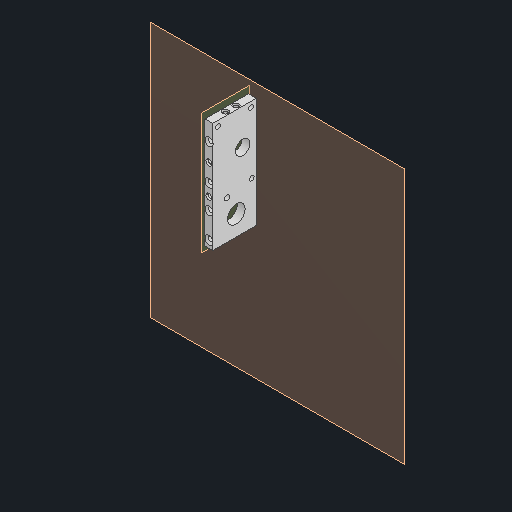
# Autodesk Inventor part: right_gear_holder
Saved by Autodesk Inventor 2023 (Build 270158000, 158)
## iProperties
Created: 2024-04-23
Part Number: right_gear_holder
Material: Generic
Document SubType Name: Modeling
Designer: szymo
Density: 1 g/cm^3
Appearance: Default
Author: szymo
Autodesk Inventor part; units mm, degrees
ref_plane "YZ Plane" through (0, 0, 0) normal (1, 0, 0) x (0, 1, 0)
ref_plane "XZ Plane" through (0, 0, 0) normal (0, 1, 0) x (-1, 0, 0)
ref_plane "Work Plane1" through (0, 0, 0) normal (0, 0, 1) x (1, 0, 0)
sketch "Sketch1" plane through (0, 0, 0) normal (0, 0, 1) x (1, 0, 0)
  line L0 (23.5, 88.5) -> (-23.5, 88.5) projected
  line L1 (-23.5, 88.5) -> (-23.5, 36.5) projected
  line L2 (-26.5, 33.5) -> (-89, 33.5) projected
  line L3 (-89, 33.5) -> (-89, -72.5) projected
  line L4 (-89, -72.5) -> (-77, -72.5) projected
  line L5 (-74, -75.5) -> (-74, -93.5) projected
  line L6 (-74, -93.5) -> (74, -93.5) projected
  line L7 (74, -93.5) -> (74, -75.5) projected
  line L8 (77, -72.5) -> (89, -72.5) projected
  line L9 (89, -72.5) -> (89, 33.5) projected
  line L10 (89, 33.5) -> (26.5, 33.5) projected
  line L11 (23.5, 36.5) -> (23.5, 88.5) projected
  line L12 (-4.5, 81.5) -> (-4.5, 36.5) projected
  line L13 (-7.5, 33.5) -> (-13.5, 33.5) projected
  line L14 (-16.5, 36.5) -> (-16.5, 81.5) projected
  line L15 (-13.5, 84.5) -> (-7.5, 84.5) projected
  line L16 (16.5, 81.5) -> (16.5, 36.5) projected
  line L17 (13.5, 33.5) -> (7.5, 33.5) projected
  line L18 (4.5, 36.5) -> (4.5, 81.5) projected
  line L19 (7.5, 84.5) -> (13.5, 84.5) projected
  line L20 (-16.5, 88.5) -> (-22.5, 88.5)
  line L21 (-22.5, 88.5) -> (-22.5, 3.75)
  line L22 (-22.5, 3.75) -> (-16.5, 3.75)
  line L23 (-16.5, 3.75) -> (-16.5, 88.5)
  line L24 (-32.2, 4.75) -> (-59.9, 4.75)
  arc A0 (13.5, 33.5) -> (16.5, 36.5) centre (13.5, 36.5) ccw projected
  arc A1 (4.5, 36.5) -> (7.5, 33.5) centre (7.5, 36.5) ccw projected
  arc A2 (7.5, 84.5) -> (4.5, 81.5) centre (7.5, 81.5) ccw projected
  arc A3 (16.5, 81.5) -> (13.5, 84.5) centre (13.5, 81.5) ccw projected
  arc A4 (-4.5, 81.5) -> (-7.5, 84.5) centre (-7.5, 81.5) ccw projected
  arc A5 (-7.5, 33.5) -> (-4.5, 36.5) centre (-7.5, 36.5) ccw projected
  arc A6 (-16.5, 36.5) -> (-13.5, 33.5) centre (-13.5, 36.5) ccw projected
  arc A7 (-13.5, 84.5) -> (-16.5, 81.5) centre (-13.5, 81.5) ccw projected
  arc A8 (-26.5, 33.5) -> (-23.5, 36.5) centre (-26.5, 36.5) ccw projected
  arc A9 (-74, -75.5) -> (-77, -72.5) centre (-77, -75.5) ccw projected
  arc A10 (77, -72.5) -> (74, -75.5) centre (77, -75.5) ccw projected
  arc A11 (23.5, 36.5) -> (26.5, 33.5) centre (26.5, 36.5) ccw projected
  point P0 (0, 0)
  point P1 (-16.5, 36.5)
  point P2 (-16.5, 81.5)
  dimension "d0" = 1
  dimension "d2" = 1
  constraints: 10 end point, 2 horizontal, 2 parallel, 1 collinear, 1 perpendicular, 1 point on line, 2 other
  measures "d0" distance between parallel lines of L1 L21
  measures "d2" distance between parallel lines of L24 L22
ref_plane "Work Plane2" through (-89, -40.3889, 33.5) normal (0, 0, 1) x (1, 0, 0)
extrude "Extrusion1" add sketch "Sketch1" along normal up to surface (33.5 mm away) contours L23 L14 L22 L21 L0
sketch "Sketch2" plane through (-22.5, 3.75, 0) normal (-1, 0, 0) x (0, 0, 1)
  arc A0 (13.7043, 9.7757) -> (14.863, 11.545) centre (10.3771, 13.2188) ccw projected
  arc A1 (14.863, 11.545) -> (15.4685, 11.512) centre (15.375, 15.375) ccw projected
  arc A2 (15.4685, 11.512) -> (16.4285, 9.6275) centre (20.1095, 12.6893) ccw projected
  arc A3 (16.4285, 9.6275) -> (17.3146, 9.863) centre (15.375, 15.375) ccw projected
  arc A4 (17.3146, 9.863) -> (17.2121, 11.9755) centre (12.599, 10.6929) ccw projected
  arc A5 (17.2121, 11.9755) -> (17.7212, 12.3047) centre (15.375, 15.375) ccw projected
  arc A6 (17.7212, 12.3047) -> (19.6056, 11.3444) centre (20.7839, 15.9851) ccw projected
  arc A7 (19.6056, 11.3444) -> (20.184, 12.0558) centre (15.375, 15.375) ccw projected
  arc A8 (20.184, 12.0558) -> (18.8594, 13.7045) centre (15.8813, 9.9554) ccw projected
  arc A9 (18.8594, 13.7045) -> (19.0778, 14.2702) centre (15.375, 15.375) ccw projected
  arc A10 (19.0778, 14.2702) -> (21.1668, 14.6008) centre (19.3923, 19.0479) ccw projected
  arc A11 (21.1668, 14.6008) -> (21.2166, 15.5164) centre (15.375, 15.375) ccw projected
  arc A12 (21.2166, 15.5164) -> (19.1758, 16.0716) centre (18.9701, 11.288) ccw projected
  arc A13 (19.1758, 16.0716) -> (19.02, 16.6576) centre (15.375, 15.375) ccw projected
  arc A14 (19.02, 16.6576) -> (20.5157, 18.153) centre (16.4662, 20.7077) ccw projected
  arc A15 (20.5157, 18.153) -> (20.0178, 18.923) centre (15.375, 15.375) ccw projected
  arc A16 (20.0178, 18.923) -> (18.0404, 18.1726) centre (20.6858, 14.1817) ccw projected
  arc A17 (18.0404, 18.1726) -> (17.57, 18.5552) centre (15.375, 15.375) ccw projected
  arc A18 (17.57, 18.5552) -> (17.9011, 20.644) centre (13.1233, 20.3306) ccw projected
  arc A19 (17.9011, 20.644) -> (17.0457, 20.9743) centre (15.375, 15.375) ccw projected
  arc A20 (17.0457, 20.9743) -> (15.887, 19.205) centre (20.3729, 17.5312) ccw projected
  arc A21 (15.887, 19.205) -> (15.2815, 19.238) centre (15.375, 15.375) ccw projected
  arc A22 (15.2815, 19.238) -> (14.3215, 21.1225) centre (10.6405, 18.0607) ccw projected
  arc A23 (14.3215, 21.1225) -> (13.4354, 20.887) centre (15.375, 15.375) ccw projected
  arc A24 (13.4354, 20.887) -> (13.5379, 18.7745) centre (18.151, 20.0571) ccw projected
  arc A25 (13.5379, 18.7745) -> (13.0288, 18.4453) centre (15.375, 15.375) ccw projected
  arc A26 (13.0288, 18.4453) -> (11.1444, 19.4056) centre (9.9661, 14.7649) ccw projected
  arc A27 (11.1444, 19.4056) -> (10.566, 18.6942) centre (15.375, 15.375) ccw projected
  arc A28 (10.566, 18.6942) -> (11.8906, 17.0455) centre (14.8687, 20.7946) ccw projected
  arc A29 (11.8906, 17.0455) -> (11.6722, 16.4798) centre (15.375, 15.375) ccw projected
  arc A30 (11.6722, 16.4798) -> (9.5832, 16.1492) centre (11.3577, 11.7021) ccw projected
  arc A31 (9.5832, 16.1492) -> (9.5334, 15.2336) centre (15.375, 15.375) ccw projected
  arc A32 (9.5334, 15.2336) -> (11.5742, 14.6784) centre (11.7799, 19.462) ccw projected
  arc A33 (11.5742, 14.6784) -> (11.73, 14.0924) centre (15.375, 15.375) ccw projected
  arc A34 (11.73, 14.0924) -> (10.2343, 12.597) centre (14.2838, 10.0423) ccw projected
  arc A35 (10.2343, 12.597) -> (10.7322, 11.827) centre (15.375, 15.375) ccw projected
  arc A36 (10.7322, 11.827) -> (12.7096, 12.5774) centre (10.0642, 16.5683) ccw projected
  arc A37 (12.7096, 12.5774) -> (13.18, 12.1948) centre (15.375, 15.375) ccw projected
  arc A38 (13.18, 12.1948) -> (12.8489, 10.106) centre (17.6267, 10.4194) ccw projected
  arc A39 (12.8489, 10.106) -> (13.7043, 9.7757) centre (15.375, 15.375) ccw projected
  circle A40 centre (15.375, 15.375) radius 6.75
  circle A41 centre (15.375, 15.375) radius 5.8433
  line L0 (21.2183, 15.375) -> (22.125, 15.375)
  circle A42 centre (10.5, 57.25) radius 5.5 projected
  point P0 (0, -3.75)
  dimension "d6" = 13.5
  dimension "d5" = 0.9067
  dimension "d9" = 11
  constraints: 3 horizontal, 2 coincident, 2 end point, 2 horizontal alignment, 5 other
  measures "d5" distance of L0.start L0.end
  measures "d9" diameter of A42
extrude "Extrusion2" cut sketch "Sketch2" against normal up to next contours A39 A38 A37 A36 A35 A34 A33 A32 A31 A30 A29 A28 A27 A26 A25 A24 A23 A22 A21 A20 A19 A18 A17 A16 A15 A14 A13 A12 A11 A10 A9 A8 A7 A6 A5 A4 A3 A2 A1 A0 | A0 A1 A2 A41 | A41 A36 A37 A38 | A4 A5 A6 A41 | A41 A32 A33 A34 | A8 A9 A10 A41 | A41 A28 A29 A30 | A41 A24 A25 A26 | A12 A13 A14 A41 | A41 A20 A21 A22 | A16 A17 A18 A41 | A40 | A42
sketch "Sketch3" plane through (-16.5, 3.75, 0) normal (1, 0, 0) x (0, 0, -1)
  circle A0 centre (-22.4424, 29.7295) radius 2 projected
  point P0 (0, -3.75)
extrude "Extrusion3" cut sketch "Sketch3" against normal blind 5
ref_plane "Work Plane3" through (-23.5, 3.75, 0) normal (-1, 0, 0) x (0, 0, 1)
sketch "Sketch5" plane through (-23.5, 3.75, 0) normal (-1, 0, 0) x (0, 0, 1)
  circle A0 centre (29.5, 80.75) radius 2.1 projected
  circle A1 centre (4, 80.75) radius 2.1 projected
  circle A2 centre (3.5, 33.25) radius 2.1 projected
  point P0 (0, -3.75)
hole "Hole1" at (-23.5, 84.5, 29.5) at (-23.5, 84.5, 4) at (-23.5, 37, 3.5) direction (1, 0, 0) diameter 3.6 end through all countersink diameter 6.2 countersink angle 90 clearance for "Countersunk Flat Head Screw ISO 2009/7046" size "M3" standard "ISO"
sketch "Sketch6" plane through (-22.5, 3.75, 33.5) normal (0, 0, 1) x (1, 0, 0)
  line L0 (0, 8.625) -> (0, 22.125) projected
  line L1 (1, 31.7295) -> (1, 27.7295) projected
  line L2 (0, 31.15) -> (0, 35.35) projected
  line L3 (0, 51.75) -> (0, 62.75) projected
  line L4 (0, 78.65) -> (0, 82.85) projected
  line L5 (0, 78.65) -> (0, 82.85) projected
  line L6 (6, 0) -> (0, 0) projected
  line L7 (6, 84.75) -> (6, 0) projected
  line L8 (0, 84.75) -> (6, 84.75) projected
  line L9 (0, 0) -> (0, 84.75) projected
  line L10 (6, 28.125) -> (0, 28.125)
  line L11 (0, 28.125) -> (0, 35.35)
  line L12 (0, 35.35) -> (6, 35.35)
  line L13 (6, 35.35) -> (6, 28.125)
  line L14 (0, 8.625) -> (6, 8.625) projected
  line L15 (6, 8.625) -> (0, 8.625)
  line L16 (0, 8.625) -> (0, 22.125)
  line L17 (0, 22.125) -> (6, 22.125)
  line L18 (6, 22.125) -> (6, 8.625)
  line L19 (6, 78.95) -> (0.3, 78.95) projected
  line L20 (6, 84.75) -> (0, 84.75) projected
  line L21 (6, 78.95) -> (0, 78.95)
  line L22 (0, 78.95) -> (0, 84.75)
  line L23 (0, 84.75) -> (6, 84.75)
  line L24 (6, 84.75) -> (6, 78.95)
  line L25 (0, 51.75) -> (6, 51.75) projected
  line L26 (0, 51.75) -> (0, 62.75) projected
  line L27 (6, 51.75) -> (0, 51.75)
  line L28 (0, 51.75) -> (0, 62.75)
  line L29 (0, 62.75) -> (6, 62.75)
  line L30 (6, 62.75) -> (6, 51.75)
  line L31 (6, 0) -> (0, 0)
  line L32 (0, 0) -> (0, 3.7)
  line L33 (0, 3.7) -> (6, 3.7)
  line L34 (6, 3.7) -> (6, 0)
  circle A0 centre (3, 5.5) radius 1.8
  line L35 (6, 22.125) -> (0, 28.125)
  line L36 (0, 22.125) -> (6, 28.125)
  line L37 (6, 35.35) -> (0, 51.75)
  line L38 (0, 35.35) -> (6, 51.75)
  line L39 (0.3, 82.55) -> (0.3, 78.95) projected
  line L40 (6, 62.75) -> (0.3, 78.95)
  line L41 (6, 82.55) -> (6, 78.95) projected
  line L42 (0.3, 78.95) -> (6, 78.95)
  line L43 (6, 78.95) -> (0, 62.75)
  point P0 (22.5, -3.75)
  point P1 (3, 25.125)
  point P2 (3.0769, 71.0577)
  point P3 (3, 43.55)
  dimension "d20" = 3.7
  dimension "d21" = 3.6
  dimension "d22" = 3
  dimension "d23" = 3
  constraints: 54 end point, 10 parallel, 7 perpendicular, 6 point on line, 5 horizontal, 2 midpoint, 1 centre point, 1 coincident, 1 tangent, 5 other
  measures "d20" distance of L31.end L32.end
  measures "d21" diameter of A0
  measures "d23" distance from line of A0.centre L9
hole "Hole2" at (-19.5, 28.875, 33.5) at (-19.5, 9.25, 33.5) at (-19.4231, 74.8077, 33.5) at (-19.5, 47.3, 33.5) direction (0, 0, -1) diameter 3.6 end through all countersink diameter 6.3 countersink angle 90 clearance for "Countersunk Flat Head Screw ISO 2009/7046" size "M3" standard "ISO"
sketch "Sketch7" plane through (-22.5, 3.75, 0) normal (0, -1, 0) x (1, 0, 0)
  line L0 (6, 33.5) -> (0, 33.5) projected
  line L1 (0, 0) -> (0, 33.5) projected
  line L2 (0, 0) -> (6, 0) projected
  line L3 (6, 0) -> (6, 33.5) projected
  line L4 (0, 0) -> (0, 33.5) projected
  line L5 (0, 16.75) -> (6, 16.75)
  line L6 (6, 16.75) -> (0, 33.5)
  line L7 (6, 16.75) -> (0, 0)
  line L8 (6, 0) -> (0, 0) projected
  line L9 (6, 0) -> (0, 16.75)
  line L10 (0, 33.5) -> (6, 33.5) projected
  line L11 (6, 33.5) -> (0, 16.75)
  point P0 (22.5, 0)
  point P1 (3, 25.125)
  point P2 (3, 8.375)
  constraints: 10 end point, 4 midpoint
hole "Hole3" at (-19.5, 3.75, 25.125) at (-19.5, 3.75, 8.375) direction (0, 1, 0) diameter 4 depth 3.6 counterbore diameter 4.6 counterbore depth 0.6
sketch "Sketch9" plane through (-22.5, 88.5, 0) normal (0, 1, 0) x (1, 0, 0)
  circle A0 centre (22.5, -20.825) radius 2.3 projected
  circle A1 centre (22.5, -12.675) radius 2.3 projected
  line L0 (18, -33.5) -> (27, -33.5) projected
  line L1 (27, 0) -> (27, -33.5) projected
  line L2 (27, 0) -> (18, 0) projected
  line L3 (18, 0) -> (18, -33.5) projected
  line L4 (22.5, -20.825) -> (0, -20.825)
  line L5 (0, -22.125) -> (0, -8.625) projected
  line L6 (22.5, -12.675) -> (0, -12.675)
  line L7 (6, 0) -> (6, -33.5) projected
  point P0 (22.5, 0)
  point P1 (3, -20.825)
  point P2 (3, -12.675)
  dimension "d45" = 3
  dimension "d46" = 3
  dimension "d47" = 3
  dimension "d48" = 3
  constraints: 4 end point, 4 point on line, 1 horizontal, 1 perpendicular
  measures "d45" distance from line of point (3, -20.825) L5
  measures "d46" distance from line of L7 point (3, -20.825)
  measures "d47" distance from line of L7 point (3, -12.675)
  measures "d48" distance from line of point (3, -12.675) L5
hole "Hole5" at (-19.5, 88.5, 20.825) at (-19.5, 88.5, 12.675) direction (0, -1, 0) diameter 4 depth 6 counterbore diameter 4.6 counterbore depth 1.5
sketch "Sketch10" plane through (-19.5, 47.3, 33.5) normal (0, 0, 1) x (1, 0, 0)
  line L0 (-3, 8.2) -> (-3, 19.2) projected
  arc A0 (3, -17.4645) -> (-3, -17.4645) centre (0, -18.425) ccw projected
  arc A1 (-3, -0.9605) -> (3, -0.9605) centre (0, 0) ccw projected
  arc A2 (3, -17.4645) -> (-3, -17.4645) centre (0, -18.425) ccw projected
  line L1 (3, -0.9605) -> (3, -17.4645) projected
  arc A3 (-3, -0.9605) -> (3, -0.9605) centre (0, 0) ccw projected
  line L2 (-3, -17.4645) -> (-3, -0.9605) projected
  line L3 (3, 8.2) -> (-3, 8.2)
  line L4 (3, 19.2) -> (-3, 19.2)
  line L5 (-3, 19.2) -> (3, 8.2)
  line L6 (-3, 8.2) -> (3, 19.2)
  line L7 (3, -17.4645) -> (-3, -0.9605)
  line L8 (-3, -17.4645) -> (3, -0.9605)
  point P0 (19.5, -47.3)
  point P1 (0, -9.2125)
  point P2 (0, 13.7)
  constraints: 12 end point, 2 horizontal, 2 midpoint, 2 other
hole "Hole6" at (-19.5, 38.0875, 33.5) at (-19.5, 61, 33.5) direction (0, 0, -1) diameter 4 depth 6 counterbore diameter 4.6 counterbore depth 1.5
equation "\"d22\" = d23"
equation "\"d45\" = d46"
equation "\"d47\" = d48"
body "Solid1"
